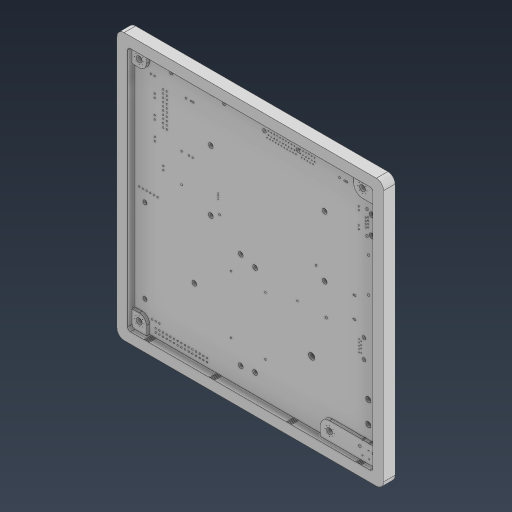
# Autodesk Inventor part: base
Saved by Autodesk Inventor 2024.2 (Build 282272000, 272)
## iProperties
Created: 2024-04-12
Part Number: base
Material: 一般
Document SubType Name: Modeling
Designer: pomelo
Density: 1 g/cm^3
Appearance: 預設
Author: pomelo
Autodesk Inventor part; units mm, degrees
ref_plane "YZ Plane" through (0, 0, 0) normal (1, 0, 0) x (0, 1, 0)
ref_plane "XZ Plane" through (0, 0, 0) normal (0, 1, 0) x (-1, 0, 0)
ref_plane "XY Plane" through (0, 0, 0) normal (0, 0, 1) x (1, 0, 0)
ref_plane "工作平面1" through (57.158, 77.35, -8.56) normal (0, 0, -1) x (-1, 0, 0)
sketch "草圖1" plane through (57.158, 77.35, -8.56) normal (0, 0, -1) x (-1, 0, 0)
  arc A0 (114.819, -181.83) -> (114.319, -181.83) centre (114.569, -181.83) ccw
  line L0 (115.129, -181.83) -> (114.819, -181.83)
  arc A1 (115.629, -181.83) -> (115.129, -181.83) centre (115.379, -181.83) ccw
  line L1 (124.759, -181.83) -> (115.629, -181.83)
  arc A2 (124.759, -181.83) -> (126.759, -179.83) centre (124.759, -179.83) ccw
  line L2 (126.759, -13.65) -> (126.759, -179.83)
  arc A3 (126.759, -13.65) -> (124.759, -11.65) centre (124.759, -13.65) ccw
  line L3 (115.629, -11.65) -> (124.759, -11.65)
  arc A4 (115.129, -11.65) -> (115.629, -11.65) centre (115.379, -11.65) ccw
  line L4 (114.819, -11.65) -> (115.129, -11.65)
  arc A5 (114.319, -11.65) -> (114.819, -11.65) centre (114.569, -11.65) ccw
  line L5 (114.009, -11.65) -> (114.319, -11.65)
  arc A6 (113.509, -11.65) -> (114.009, -11.65) centre (113.759, -11.65) ccw
  line L6 (113.199, -11.65) -> (113.509, -11.65)
  arc A7 (112.699, -11.65) -> (113.199, -11.65) centre (112.949, -11.65) ccw
  line L7 (112.389, -11.65) -> (112.699, -11.65)
  arc A8 (111.889, -11.65) -> (112.389, -11.65) centre (112.139, -11.65) ccw
  line L8 (70.236, -11.65) -> (111.889, -11.65)
  arc A9 (69.736, -11.65) -> (70.236, -11.65) centre (69.986, -11.65) ccw
  line L9 (69.426, -11.65) -> (69.736, -11.65)
  arc A10 (68.926, -11.65) -> (69.426, -11.65) centre (69.176, -11.65) ccw
  line L10 (68.616, -11.65) -> (68.926, -11.65)
  arc A11 (68.116, -11.65) -> (68.616, -11.65) centre (68.366, -11.65) ccw
  line L11 (67.806, -11.65) -> (68.116, -11.65)
  arc A12 (67.306, -11.65) -> (67.806, -11.65) centre (67.556, -11.65) ccw
  line L12 (66.996, -11.65) -> (67.306, -11.65)
  arc A13 (66.496, -11.65) -> (66.996, -11.65) centre (66.746, -11.65) ccw
  line L13 (16.842, -11.65) -> (66.496, -11.65)
  arc A14 (16.342, -11.65) -> (16.842, -11.65) centre (16.592, -11.65) ccw
  line L14 (16.032, -11.65) -> (16.342, -11.65)
  arc A15 (15.532, -11.65) -> (16.032, -11.65) centre (15.782, -11.65) ccw
  line L15 (15.222, -11.65) -> (15.532, -11.65)
  arc A16 (14.722, -11.65) -> (15.222, -11.65) centre (14.972, -11.65) ccw
  line L16 (14.412, -11.65) -> (14.722, -11.65)
  arc A17 (13.912, -11.65) -> (14.412, -11.65) centre (14.162, -11.65) ccw
  line L17 (13.602, -11.65) -> (13.912, -11.65)
  arc A18 (13.102, -11.65) -> (13.602, -11.65) centre (13.352, -11.65) ccw
  line L18 (-31.551, -11.65) -> (13.102, -11.65)
  arc A19 (-32.051, -11.65) -> (-31.551, -11.65) centre (-31.801, -11.65) ccw
  line L19 (-32.361, -11.65) -> (-32.051, -11.65)
  arc A20 (-32.861, -11.65) -> (-32.361, -11.65) centre (-32.611, -11.65) ccw
  line L20 (-33.171, -11.65) -> (-32.861, -11.65)
  arc A21 (-33.671, -11.65) -> (-33.171, -11.65) centre (-33.421, -11.65) ccw
  line L21 (-33.981, -11.65) -> (-33.671, -11.65)
  arc A22 (-34.481, -11.65) -> (-33.981, -11.65) centre (-34.231, -11.65) ccw
  line L22 (-34.791, -11.65) -> (-34.481, -11.65)
  arc A23 (-35.291, -11.65) -> (-34.791, -11.65) centre (-35.041, -11.65) ccw
  line L23 (-41.421, -11.65) -> (-35.291, -11.65)
  arc A24 (-41.421, -11.65) -> (-43.421, -13.65) centre (-41.421, -13.65) ccw
  line L24 (-43.421, -179.83) -> (-43.421, -13.65)
  arc A25 (-43.421, -179.83) -> (-41.421, -181.83) centre (-41.421, -179.83) ccw
  line L25 (-35.291, -181.83) -> (-41.421, -181.83)
  arc A26 (-34.791, -181.83) -> (-35.291, -181.83) centre (-35.041, -181.83) ccw
  line L26 (-34.481, -181.83) -> (-34.791, -181.83)
  arc A27 (-33.981, -181.83) -> (-34.481, -181.83) centre (-34.231, -181.83) ccw
  line L27 (-33.671, -181.83) -> (-33.981, -181.83)
  arc A28 (-33.171, -181.83) -> (-33.671, -181.83) centre (-33.421, -181.83) ccw
  line L28 (-32.861, -181.83) -> (-33.171, -181.83)
  arc A29 (-32.361, -181.83) -> (-32.861, -181.83) centre (-32.611, -181.83) ccw
  line L29 (-32.051, -181.83) -> (-32.361, -181.83)
  arc A30 (-31.551, -181.83) -> (-32.051, -181.83) centre (-31.801, -181.83) ccw
  line L30 (13.102, -181.83) -> (-31.551, -181.83)
  arc A31 (13.602, -181.83) -> (13.102, -181.83) centre (13.352, -181.83) ccw
  line L31 (13.912, -181.83) -> (13.602, -181.83)
  arc A32 (14.412, -181.83) -> (13.912, -181.83) centre (14.162, -181.83) ccw
  line L32 (14.722, -181.83) -> (14.412, -181.83)
  arc A33 (15.222, -181.83) -> (14.722, -181.83) centre (14.972, -181.83) ccw
  line L33 (15.532, -181.83) -> (15.222, -181.83)
  arc A34 (16.032, -181.83) -> (15.532, -181.83) centre (15.782, -181.83) ccw
  line L34 (16.342, -181.83) -> (16.032, -181.83)
  arc A35 (16.842, -181.83) -> (16.342, -181.83) centre (16.592, -181.83) ccw
  line L35 (66.496, -181.83) -> (16.842, -181.83)
  arc A36 (66.996, -181.83) -> (66.496, -181.83) centre (66.746, -181.83) ccw
  line L36 (67.306, -181.83) -> (66.996, -181.83)
  arc A37 (67.806, -181.83) -> (67.306, -181.83) centre (67.556, -181.83) ccw
  line L37 (68.116, -181.83) -> (67.806, -181.83)
  arc A38 (68.616, -181.83) -> (68.116, -181.83) centre (68.366, -181.83) ccw
  line L38 (68.926, -181.83) -> (68.616, -181.83)
  arc A39 (69.426, -181.83) -> (68.926, -181.83) centre (69.176, -181.83) ccw
  line L39 (69.736, -181.83) -> (69.426, -181.83)
  arc A40 (70.236, -181.83) -> (69.736, -181.83) centre (69.986, -181.83) ccw
  line L40 (111.889, -181.83) -> (70.236, -181.83)
  arc A41 (112.389, -181.83) -> (111.889, -181.83) centre (112.139, -181.83) ccw
  line L41 (112.699, -181.83) -> (112.389, -181.83)
  arc A42 (113.199, -181.83) -> (112.699, -181.83) centre (112.949, -181.83) ccw
  line L42 (113.509, -181.83) -> (113.199, -181.83)
  arc A43 (114.009, -181.83) -> (113.509, -181.83) centre (113.759, -181.83) ccw
  line L43 (114.319, -181.83) -> (114.009, -181.83)
  line L44 (-25.056, -101.2) -> (-26.256, -101.2)
  arc A44 (-25.056, -102.1) -> (-25.056, -101.2) centre (-25.056, -101.65) ccw
  line L45 (-26.256, -102.1) -> (-25.056, -102.1)
  arc A45 (-26.256, -101.2) -> (-26.256, -102.1) centre (-26.256, -101.65) ccw
  line L46 (-40.296, -86.7) -> (-40.996, -86.7)
  arc A46 (-40.296, -87.6) -> (-40.296, -86.7) centre (-40.296, -87.15) ccw
  line L47 (-40.996, -87.6) -> (-40.296, -87.6)
  arc A47 (-40.996, -86.7) -> (-40.996, -87.6) centre (-40.996, -87.15) ccw
  line L48 (-25.056, -86.7) -> (-26.256, -86.7)
  arc A48 (-25.056, -87.6) -> (-25.056, -86.7) centre (-25.056, -87.15) ccw
  line L49 (-26.256, -87.6) -> (-25.056, -87.6)
  arc A49 (-26.256, -86.7) -> (-26.256, -87.6) centre (-26.256, -87.15) ccw
  line L50 (-40.296, -101.2) -> (-40.996, -101.2)
  arc A50 (-40.296, -102.1) -> (-40.296, -101.2) centre (-40.296, -101.65) ccw
  line L51 (-40.996, -102.1) -> (-40.296, -102.1)
  arc A51 (-40.996, -101.2) -> (-40.996, -102.1) centre (-40.996, -101.65) ccw
  circle A52 centre (119.679, -104) radius 1.375
  circle A53 centre (119.679, -162) radius 1.375
  circle A54 centre (-35.321, -145) radius 1.75
  circle A55 centre (-35.321, -160) radius 1.75
  circle A56 centre (0.96, -82.55) radius 0.635
  circle A57 centre (68.04, -85.6) radius 0.635
  circle A58 centre (13.978, -110.374) radius 0.55
  circle A59 centre (-6.02, -110.374) radius 0.8
  circle A60 centre (-5, -47) radius 1.6
  circle A61 centre (74, -89) radius 1.6
  circle A62 centre (-5, -89) radius 1.6
  circle A63 centre (74, -47) radius 1.6
  circle A64 centre (43.279, -105) radius 1.6
  circle A65 centre (53.211, -102) radius 1.6
  circle A66 centre (53.211, -169) radius 1.6
  circle A67 centre (43.279, -168) radius 1.6
  circle A68 centre (85.411, -135.5) radius 1.6
  circle A69 centre (86.61, -60.633) radius 0.51
  circle A70 centre (89.15, -60.633) radius 0.51
  circle A71 centre (112.879, -63.865) radius 0.51
  circle A72 centre (112.879, -61.325) radius 0.51
  circle A73 centre (107.004, -75.735) radius 0.51
  circle A74 centre (107.004, -78.275) radius 0.51
  circle A75 centre (115.594, -24.725) radius 0.51
  circle A76 centre (113.054, -24.725) radius 0.51
  circle A77 centre (112.979, -37.84) radius 0.51
  circle A78 centre (112.979, -35.3) radius 0.51
  circle A79 centre (112.979, -50.84) radius 0.51
  circle A80 centre (112.979, -48.3) radius 0.51
  circle A81 centre (64.679, -17.2) radius 1.05
  circle A82 centre (101.479, -17.2) radius 1.05
  circle A83 centre (94.309, -80.765) radius 0.545
  circle A84 centre (94.309, -60.635) radius 0.545
  circle A85 centre (107.119, -52.7) radius 0.51
  circle A86 centre (107.119, -50.16) radius 0.51
  circle A87 centre (107.119, -47.62) radius 0.51
  circle A88 centre (107.119, -45.08) radius 0.51
  circle A89 centre (107.119, -42.54) radius 0.51
  circle A90 centre (107.119, -40) radius 0.51
  circle A91 centre (107.119, -37.46) radius 0.51
  circle A92 centre (107.119, -34.92) radius 0.51
  circle A93 centre (107.119, -32.38) radius 0.51
  circle A94 centre (107.119, -29.84) radius 0.51
  circle A95 centre (104.579, -52.7) radius 0.51
  circle A96 centre (104.579, -50.16) radius 0.51
  circle A97 centre (104.579, -47.62) radius 0.51
  circle A98 centre (104.579, -45.08) radius 0.51
  circle A99 centre (104.579, -42.54) radius 0.51
  circle A100 centre (104.579, -40) radius 0.51
  circle A101 centre (104.579, -37.46) radius 0.51
  circle A102 centre (104.579, -34.92) radius 0.51
  circle A103 centre (104.579, -32.38) radius 0.51
  circle A104 centre (104.579, -29.84) radius 0.51
  circle A105 centre (121.679, -175.48) radius 1.975
  circle A106 centre (119.398, -177.761) radius 0.175
  circle A107 centre (121.679, -178.706) radius 0.175
  circle A108 centre (123.96, -177.761) radius 0.175
  circle A109 centre (124.905, -175.48) radius 0.175
  circle A110 centre (123.96, -173.199) radius 0.175
  circle A111 centre (121.679, -172.254) radius 0.175
  circle A112 centre (119.398, -173.199) radius 0.175
  circle A113 centre (118.453, -175.48) radius 0.175
  circle A114 centre (121.679, -18) radius 1.975
  circle A115 centre (119.398, -20.281) radius 0.175
  circle A116 centre (121.679, -21.226) radius 0.175
  circle A117 centre (123.96, -20.281) radius 0.175
  circle A118 centre (124.905, -18) radius 0.175
  circle A119 centre (123.96, -15.719) radius 0.175
  circle A120 centre (121.679, -14.774) radius 0.175
  circle A121 centre (119.398, -15.719) radius 0.175
  circle A122 centre (118.453, -18) radius 0.175
  circle A123 centre (-10.401, -175.48) radius 1.975
  circle A124 centre (-12.682, -177.761) radius 0.175
  circle A125 centre (-10.401, -178.706) radius 0.175
  circle A126 centre (-8.12, -177.761) radius 0.175
  circle A127 centre (-7.175, -175.48) radius 0.175
  circle A128 centre (-8.12, -173.199) radius 0.175
  circle A129 centre (-10.401, -172.254) radius 0.175
  circle A130 centre (-12.682, -173.199) radius 0.175
  circle A131 centre (-13.627, -175.48) radius 0.175
  circle A132 centre (-33.241, -18) radius 1.975
  circle A133 centre (-35.522, -20.281) radius 0.175
  circle A134 centre (-33.241, -21.226) radius 0.175
  circle A135 centre (-30.96, -20.281) radius 0.175
  circle A136 centre (-30.015, -18) radius 0.175
  circle A137 centre (-30.96, -15.719) radius 0.175
  circle A138 centre (-33.241, -14.774) radius 0.175
  circle A139 centre (-35.522, -15.719) radius 0.175
  circle A140 centre (-36.467, -18) radius 0.175
  circle A141 centre (112.239, -178.54) radius 0.51
  circle A142 centre (112.239, -176) radius 0.51
  circle A143 centre (109.699, -178.54) radius 0.51
  circle A144 centre (109.699, -176) radius 0.51
  circle A145 centre (107.159, -178.54) radius 0.51
  circle A146 centre (107.159, -176) radius 0.51
  circle A147 centre (104.619, -178.54) radius 0.51
  circle A148 centre (104.619, -176) radius 0.51
  circle A149 centre (102.079, -178.54) radius 0.51
  circle A150 centre (102.079, -176) radius 0.51
  circle A151 centre (99.539, -178.54) radius 0.51
  circle A152 centre (99.539, -176) radius 0.51
  circle A153 centre (96.999, -178.54) radius 0.51
  circle A154 centre (96.999, -176) radius 0.51
  circle A155 centre (94.459, -178.54) radius 0.51
  circle A156 centre (94.459, -176) radius 0.51
  circle A157 centre (91.919, -178.54) radius 0.51
  circle A158 centre (91.919, -176) radius 0.51
  circle A159 centre (89.379, -178.54) radius 0.51
  circle A160 centre (89.379, -176) radius 0.51
  circle A161 centre (86.839, -178.54) radius 0.51
  circle A162 centre (76.679, -178.54) radius 0.51
  circle A163 centre (79.219, -176) radius 0.51
  circle A164 centre (81.759, -176) radius 0.51
  circle A165 centre (86.839, -176) radius 0.51
  circle A166 centre (76.679, -176) radius 0.51
  circle A167 centre (79.219, -178.54) radius 0.51
  circle A168 centre (81.759, -178.54) radius 0.51
  circle A169 centre (84.299, -176) radius 0.51
  circle A170 centre (84.299, -178.54) radius 0.51
  circle A171 centre (91.279, -27.2) radius 0.595
  circle A172 centre (87.765, -27.2) radius 0.51
  circle A173 centre (86.279, -27.2) radius 0.595
  circle A174 centre (-15.321, -21.7) radius 0.595
  circle A175 centre (-18.835, -21.7) radius 0.51
  circle A176 centre (-20.321, -21.7) radius 0.595
  circle A177 centre (-31.421, -173.9) radius 0.85
  circle A178 centre (-37.421, -173.9) radius 0.4
  circle A179 centre (-33.221, -169.15) radius 0.4
  circle A180 centre (-37.921, -169.15) radius 0.4
  circle A181 centre (-37.921, -178.65) radius 0.4
  circle A182 centre (-33.221, -178.65) radius 0.4
  circle A183 centre (-40.671, -173.9) radius 0.825
  circle A184 centre (2.02, -18.325) radius 0.355
  circle A185 centre (3.02, -16.325) radius 0.355
  circle A186 centre (2.02, -20.825) radius 0.355
  circle A187 centre (3.02, -22.825) radius 0.355
  circle A188 centre (4.02, -18.325) radius 0.355
  circle A189 centre (6.02, -18.325) radius 0.355
  circle A190 centre (5.02, -16.325) radius 0.355
  circle A191 centre (4.02, -20.825) radius 0.355
  circle A192 centre (6.02, -20.825) radius 0.355
  circle A193 centre (5.02, -22.825) radius 0.355
  circle A194 centre (8.02, -18.325) radius 0.355
  circle A195 centre (10.02, -18.325) radius 0.355
  circle A196 centre (9.02, -16.325) radius 0.355
  circle A197 centre (7.02, -16.325) radius 0.355
  circle A198 centre (8.02, -20.825) radius 0.355
  circle A199 centre (10.02, -20.825) radius 0.355
  circle A200 centre (7.02, -22.825) radius 0.355
  circle A201 centre (9.02, -22.825) radius 0.355
  circle A202 centre (12.02, -18.325) radius 0.355
  circle A203 centre (11.02, -16.325) radius 0.355
  circle A204 centre (12.02, -20.825) radius 0.355
  circle A205 centre (11.02, -22.825) radius 0.355
  circle A206 centre (16.02, -18.325) radius 0.355
  circle A207 centre (15.02, -16.325) radius 0.355
  circle A208 centre (16.02, -20.825) radius 0.355
  circle A209 centre (15.02, -22.825) radius 0.355
  circle A210 centre (18.02, -18.325) radius 0.355
  circle A211 centre (17.02, -16.325) radius 0.355
  circle A212 centre (19.02, -16.325) radius 0.355
  circle A213 centre (18.02, -20.825) radius 0.355
  circle A214 centre (17.02, -22.825) radius 0.355
  circle A215 centre (19.02, -22.825) radius 0.355
  circle A216 centre (22.02, -18.325) radius 0.355
  circle A217 centre (20.02, -18.325) radius 0.355
  circle A218 centre (21.02, -16.325) radius 0.355
  circle A219 centre (20.02, -20.825) radius 0.355
  circle A220 centre (22.02, -20.825) radius 0.355
  circle A221 centre (21.02, -22.825) radius 0.355
  circle A222 centre (24.02, -18.325) radius 0.355
  circle A223 centre (23.02, -16.325) radius 0.355
  circle A224 centre (25.02, -16.325) radius 0.355
  circle A225 centre (24.02, -20.825) radius 0.355
  circle A226 centre (23.02, -22.825) radius 0.355
  circle A227 centre (25.02, -22.825) radius 0.355
  circle A228 centre (26.02, -18.325) radius 0.355
  circle A229 centre (28.02, -18.325) radius 0.355
  circle A230 centre (27.02, -16.325) radius 0.355
  circle A231 centre (26.02, -20.825) radius 0.355
  circle A232 centre (28.02, -20.825) radius 0.355
  circle A233 centre (27.02, -22.825) radius 0.355
  circle A234 centre (30.02, -18.325) radius 0.355
  circle A235 centre (29.02, -16.325) radius 0.355
  circle A236 centre (31.02, -16.325) radius 0.355
  circle A237 centre (30.02, -20.825) radius 0.355
  circle A238 centre (29.02, -22.825) radius 0.355
  circle A239 centre (31.02, -22.825) radius 0.355
  circle A240 centre (34.02, -18.325) radius 0.355
  circle A241 centre (32.02, -18.325) radius 0.355
  circle A242 centre (33.02, -16.325) radius 0.355
  circle A243 centre (32.02, -20.825) radius 0.355
  circle A244 centre (34.02, -20.825) radius 0.355
  circle A245 centre (33.02, -22.825) radius 0.355
  circle A246 centre (35.02, -16.325) radius 0.355
  circle A247 centre (35.02, -22.825) radius 0.355
  circle A248 centre (13.67, -19.575) radius 1.18
  circle A249 centre (36.82, -19.575) radius 1.18
  circle A250 centre (36.109, -156.568) radius 0.545
  circle A251 centre (36.109, -116.432) radius 0.545
  circle A252 centre (59.949, -115.432) radius 0.545
  circle A253 centre (59.949, -155.568) radius 0.545
  circle A254 centre (3.979, -138.624) radius 2.15
  circle A255 centre (110.979, -96.5) radius 0.51
  circle A256 centre (113.519, -96.5) radius 0.51
  circle A257 centre (118.599, -96.5) radius 0.51
  circle A258 centre (121.139, -96.5) radius 0.51
  circle A259 centre (123.679, -96.5) radius 0.51
  circle A260 centre (116.059, -96.5) radius 0.51
  circle A261 centre (-30.321, -119.4) radius 0.35
  circle A262 centre (-30.321, -116.9) radius 0.35
  circle A263 centre (-30.321, -114.9) radius 0.35
  circle A264 centre (-30.321, -112.4) radius 0.35
  circle A265 centre (-28.821, -111.9) radius 0.35
  circle A266 centre (-28.821, -113.9) radius 0.35
  circle A267 centre (-28.821, -115.9) radius 0.35
  circle A268 centre (-28.821, -117.9) radius 0.35
  circle A269 centre (-28.821, -119.9) radius 0.35
  circle A270 centre (-32.321, -122.47) radius 1.15
  circle A271 centre (-32.321, -109.33) radius 1.15
  circle A272 centre (-35.421, -58.15) radius 0.7
  circle A273 centre (-35.421, -82.15) radius 0.7
  circle A274 centre (-34.332, -47.234) radius 0.8
  circle A275 centre (-34.332, -30.978) radius 0.8
  circle A276 centre (-28.617, -45.964) radius 0.445
  circle A277 centre (-28.617, -43.678) radius 0.445
  circle A278 centre (-28.617, -34.534) radius 0.445
  circle A279 centre (-28.617, -32.248) radius 0.445
  circle A280 centre (-33.443, -42.662) radius 0.445
  circle A281 centre (-35.221, -39.614) radius 0.445
  circle A282 centre (-33.443, -40.63) radius 0.445
  circle A283 centre (-33.443, -38.598) radius 0.445
  circle A284 centre (-35.221, -37.582) radius 0.445
  circle A285 centre (-33.443, -36.566) radius 0.445
  circle A286 centre (-37.761, -32.756) radius 1.625
  circle A287 centre (-37.761, -45.456) radius 1.625
  circle A288 centre (-35.221, -35.55) radius 0.445
  circle A289 centre (-35.221, -41.646) radius 0.445
  circle A290 centre (68.937, -75.6) radius 0.32
  circle A291 centre (68.937, -76.85) radius 0.32
  circle A292 centre (68.937, -73.1) radius 0.32
  circle A293 centre (68.937, -74.35) radius 0.32
  circle A294 centre (114.779, -171.8) radius 0.51
  circle A295 centre (112.239, -171.8) radius 0.51
  circle A296 centre (109.699, -171.8) radius 0.51
  line L52 (-50.421, -163.95) -> (-50.421, -158.55)
  line L53 (-49.571, -158.55) -> (-49.571, -163.95)
  line L54 (-43.421, -156.15) -> (-43.421, -166.35)
  line L55 (-43.911, -166.35) -> (-43.911, -156.15)
  line L56 (-43.421, -139.65) -> (-43.421, -149.85)
  line L57 (-43.911, -149.85) -> (-43.911, -139.65)
  line L58 (-50.421, -147.45) -> (-50.421, -142.05)
  line L59 (-49.571, -142.05) -> (-49.571, -147.45)
  line L60 (129.169, -189.24) -> (-45.831, -189.24)
  line L61 (-50.831, -184.24) -> (-50.831, -9.24)
  line L62 (-45.831, -4.24) -> (129.169, -4.24)
  line L63 (134.169, -9.24) -> (134.169, -184.24)
  arc A297 (129.169, -189.24) -> (134.169, -184.24) centre (129.169, -184.24) ccw
  arc A298 (134.169, -9.24) -> (129.169, -4.24) centre (129.169, -9.24) ccw
  arc A299 (-45.831, -4.24) -> (-50.831, -9.24) centre (-45.831, -9.24) ccw
  arc A300 (-50.831, -184.24) -> (-45.831, -189.24) centre (-45.831, -184.24) ccw
  circle A301 centre (121.679, -175.48) radius 5.08
  line L64 (121.679, -170.4) -> (126.759, -170.4)
  line L65 (116.599, -175.48) -> (116.599, -181.83)
  circle A302 centre (121.679, -18) radius 5.08
  line L66 (116.599, -18) -> (116.599, -11.65)
  line L67 (121.679, -23.08) -> (126.759, -23.08)
  circle A303 centre (-33.241, -18) radius 6.1027
  line L68 (-33.241, -24.1027) -> (-43.421, -24.1027)
  line L69 (-27.1383, -18) -> (-27.1383, -11.65)
  circle A304 centre (-10.401, -175.48) radius 6.35
  line L70 (-10.401, -169.13) -> (-43.421, -169.13)
  line L71 (-4.051, -175.48) -> (-4.051, -181.83)
  circle A305 centre (27.02, -152) radius 1.5
  point P0 (74, -89)
  point P1 (-50.831, -4.24)
  point P2 (-50.831, -189.24)
  point P3 (134.169, -4.24)
  point P4 (41.669, -4.24)
  point P5 (41.669, -11.65)
  point P6 (-50.831, -96.74)
  point P7 (-43.421, -96.74)
  point P8 (-32.8215, -169.13)
  point P9 (-33.6205, -169.13)
  point P10 (-37.5215, -169.13)
  point P11 (-38.3205, -169.13)
  point P12 (-33.4068, -11.8996)
  point P13 (-33.421, -11.9)
  dimension "d1" = 185
  dimension "d2" = 185
  dimension "d3" = 5
  constraints: 306 centre point, 144 end point, 120 point on circle, 14 point on line, 7 perpendicular, 4 coincident, 4 midpoint, 4 tangent, 1 horizontal
  measures "d1" distance of point (-50.831, -189.24) point (-50.831, -4.24)
  measures "d2" distance of point (-50.831, -4.24) point (134.169, -4.24)
  measures "d3" radius of A297
extrude "底板" add sketch "草圖1" against normal blind 3 contours A0 L43 A43 L42 A42 L41 A41 L40 A40 L39 A39 L38 A38 L37 A37 L36 A36 L35 A35 L34 A34 L33 A33 L32 A32 L31 A31 L30 L71 A304 L70 A179 A180 L24 L68 A303 L69 L18 A18 L17 A17 L16 A16 L15 A15 L14 A14 L13 A13 L12 A12 L11 A11 L10 A10 L9 A9 L8 A8 L7 A7 L6 A6 L5 A5 L4 A4 L3 L66 A302 L67 L2 L64 A301 L65 L1 A1 L0 | L65 A301 L2 A2 L1 | A301 | L64 L2 A301 | L67 A302 L2 | A302 L66 L3 A3 L2 | A302 | L30 A304 L71 | L30 A30 L29 A29 L28 A28 L27 A27 L26 A26 L25 A25 L24 L70 A180 A179 A304 | A304 | L24 A24 L23 A23 L22 A22 L21 A21 A303 L68 | A303 | L69 A303 A21 L20 A20 L19 A19 L18 | A305
extrude "熱壓座" add sketch "草圖1" against normal blind 5 contours L65 A301 L2 A2 L1 | A301 | L64 L2 A301 | L67 A302 L2 | A302 L66 L3 A3 L2 | A302 | L30 A304 L71 | L30 A30 L29 A29 L28 A28 L27 A27 L26 A26 L25 A25 L24 L70 A180 A179 A304 | A304 | L24 A24 L23 A23 L22 A22 L21 A21 A303 L68 | A303 | L69 A303 A21 L20 A20 L19 A19 L18
extrude "擠出4" add sketch "草圖1" against normal blind 8 contours L60 A300 L61 A299 L62 A298 L63 A297
